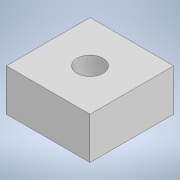
# Autodesk Inventor part: Soporte
Saved by Autodesk Inventor 2021 (Build 250183000, 183)
## iProperties
Created: 2022-01-26
Part Number: Soporte
Material: Genérico
Document SubType Name: Modeling
Designer: pc
Density: 1 g/cm^3
Appearance: Valor por defecto
Author: pc
Autodesk Inventor part; units mm, degrees
ref_plane "YZ Plane" through (0, 0, 0) normal (1, 0, 0) x (0, 1, 0)
ref_plane "XZ Plane" through (0, 0, 0) normal (0, 1, 0) x (-1, 0, 0)
ref_plane "XY Plane" through (0, 0, 0) normal (0, 0, 1) x (1, 0, 0)
sketch "Boceto1" plane through (0, 0, 0) normal (0, 1, 0) x (-1, 0, 0)
  line L0 (0, 0) -> (-1600, 0)
  line L1 (-1600, 0) -> (-1600, -1600)
  line L2 (-1600, -1600) -> (0, -1600)
  line L3 (0, -1600) -> (0, 0)
  dimension "d0" = 1600
  dimension "d1" = 1600
  constraints: 8 end point, 2 parallel, 1 horizontal, 1 perpendicular
  measures "d0" distance of L2.end L1.end
  measures "d1" distance of L1.end L0.end
extrude "Extrusión1" add sketch "Boceto1" along normal blind 800
sketch "Boceto2" plane through (0, 800, 0) normal (0, 1, 0) x (1, 0, 0)
  line L0 (0, 0) -> (800, 0)
  circle A0 centre (800, 800) radius 250
  dimension "d6" = 500
  constraints: 2 end point, 1 centre point, 1 horizontal
  measures "d6" diameter of A0
extrude "Extrusión2" cut sketch "Boceto2" against normal blind 400
